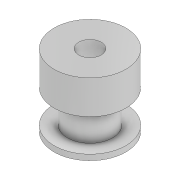
# Autodesk Inventor part: Small GT2 Belt Pully
Saved by Autodesk Inventor 2020 (Build 240168000, 168)
## iProperties
Created: 2021-02-27
Part Number: Small GT2 Belt Pully
Material: Generic
Document SubType Name: Modeling
Designer: Coy
Density: 1 g/cm^3
Appearance: Aluminum - Polished
Author: Coy
Autodesk Inventor part; units mm, degrees
ref_plane "YZ Plane" through (0, 0, 0) normal (1, 0, 0) x (0, 1, 0)
ref_plane "XZ Plane" through (0, 0, 0) normal (0, 1, 0) x (-1, 0, 0)
sketch "Sketch1" plane through (0, 0, 0) normal (0, 1, 0) x (-1, 0, 0)
  circle A0 centre (0, 0) radius 8
  circle A1 centre (0, 0) radius 2.5
  dimension "d0" = 16
  dimension "d1" = 5
  constraints: 2 centre point, 2 coincident
  measures "d0" diameter of A0
  measures "d1" diameter of A1
extrude "Extrusion1" add sketch "Sketch1" along normal blind 16
ref_plane "Work Plane1" through (0, 1.25, 0) normal (0, -1, 0) x (1, 0, 0)
sketch "Sketch2" plane through (0, 1.25, 0) normal (0, -1, 0) x (1, 0, 0)
  circle A0 centre (0, 0) radius 8 projected
  circle A1 centre (0, 0) radius 2.5 projected
  circle A2 centre (0, 0) radius 5.0201
  dimension "d5" = 2.9799
  constraints: 1 centre point
  measures "d5" radial gap between concentric circles of A0 A2
extrude "Extrusion2" cut sketch "Sketch2" against normal blind 7.25 contours A0
body "Solid1"
